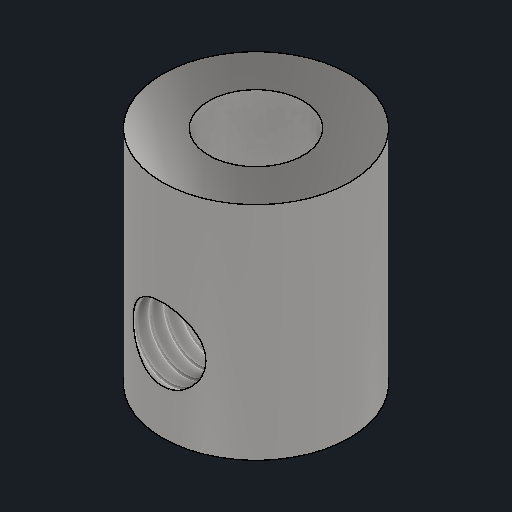
# Autodesk Inventor part: Bearing Nut
Saved by Autodesk Inventor 2026.2 (Build 302298000, 298)
## iProperties
Created: 2025-06-19
Part Number: Bearing Nut
Material: Steel, Alloy
Document SubType Name: Modeling
Designer: Joshua Eah
Density: 7.73 g/cm^3
Appearance: Semi-Polished
Author: Joshua Eah
Autodesk Inventor part; units mm, degrees
ref_plane "YZ Plane" through (0, 0, 0) normal (1, 0, 0) x (0, 1, 0)
ref_plane "XZ Plane" through (0, 0, 0) normal (0, 1, 0) x (-1, 0, 0)
sketch "Sketch1" plane through (0, 0, 0) normal (0, 1, 0) x (-1, 0, 0)
  circle A0 centre (0, 0) radius 3.175
  circle A1 centre (0, 0) radius 1.5
  dimension "d0" = 6.35
  dimension "d1" = 3
  constraints: 2 centre point, 2 coincident
  measures "d0" diameter of A0
  measures "d1" diameter of A1
extrude "Extrusion1" add sketch "Sketch1" against normal blind 7.5 contours A0 | A1
ref_plane "Work Plane1" through (0, 0, 3.175) normal (0, 0, 1) x (1, 0, 0)
sketch "Sketch2" plane through (0, 0, 3.175) normal (0, 0, 1) x (1, 0, 0)
  line L0 (-3.175, -7.5) -> (3.175, -7.5) projected
  line L1 (3.175, 0) -> (-3.175, 0) projected
  line L2 (-3.175, 0) -> (-3.175, -7.5) projected
  line L3 (-3.175, -2) -> (3.175, -2) construction
  circle A0 centre (0, -4.75) radius 1.5
  dimension "d11" = 2
  dimension "d12" = 3
  dimension "d13" = 2.75
  dimension "d14" = 3.175
  constraints: 2 end point, 1 centre point, 1 horizontal, 1 point on line
  measures "d11" distance between parallel lines of L1 L3
  measures "d12" diameter of A0
  measures "d13" distance from line of A0.centre L3
  measures "d14" distance from line of A0.centre L2
hole "Threaded Hole" at (0, -4.75, 3.175) direction (0, 0, -1) diameter 2.459 end through all thread size "M3x0.5" class "6H" standard "ANSI Metric M Profile"
hole "Pin Bearing Hole" at (0, 0, 0) direction (0, -1, 0) diameter 3.2004 depth 4.75 tip angle 118 clearance for "Socket Head Cap Screw" size "M3" standard "Ansi Metric M Profile"
equation "\"d9\" = d11 + d13"
body "Solid1"
